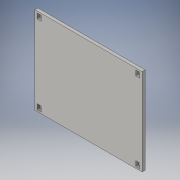
# Autodesk Inventor part: mcdave_top
Saved by Autodesk Inventor 2016 (Build 200138000, 138)
## iProperties
Created: 2017-11-29
Part Number: mcdave_top
Material: Generic
Document SubType Name: Modeling
Designer: student
Density: 1 g/cm^3
Appearance: Default
Author: student
Autodesk Inventor part; units mm, degrees
ref_plane "YZ Plane" through (0, 0, 0) normal (1, 0, 0) x (0, 1, 0)
ref_plane "XZ Plane" through (0, 0, 0) normal (0, 1, 0) x (-1, 0, 0)
ref_plane "XY Plane" through (0, 0, 0) normal (0, 0, 1) x (1, 0, 0)
sketch "Sketch1" plane through (0, 0, 0) normal (0, 0, 1) x (1, 0, 0)
  line L0 (49.1624, -46.1074) -> (-32.1176, -46.1074)
  line L1 (49.1624, -46.1074) -> (-32.1176, -46.1074)
  line L2 (-32.1176, -46.1074) -> (-32.1176, 19.9326)
  line L3 (-32.1176, -46.1074) -> (-32.1176, 19.9326)
  line L4 (49.1624, 19.9326) -> (-32.1176, 19.9326)
  line L5 (-32.1176, 19.9326) -> (49.1624, 19.9326)
  line L6 (49.1624, 19.9326) -> (49.1624, -46.1074)
  line L7 (44.3516, -40.9552) -> (47.5774, -40.9552)
  line L8 (44.3516, -40.9552) -> (47.5774, -40.9552)
  line L9 (47.5774, -40.9552) -> (47.5774, -44.8414)
  line L10 (47.5774, -40.9552) -> (47.5774, -44.8414)
  line L11 (47.5774, -44.8414) -> (44.3516, -44.8414)
  line L12 (47.5774, -44.8414) -> (44.3516, -44.8414)
  line L13 (44.3516, -44.8414) -> (44.3516, -40.9552)
  line L14 (44.3516, -44.8414) -> (44.3516, -40.9552)
  line L15 (47.5774, 14.7804) -> (47.5774, 18.6666)
  line L16 (47.5774, 14.7804) -> (44.3516, 14.7804)
  line L17 (44.3516, 14.7804) -> (44.3516, 18.6666)
  line L18 (44.3516, 14.7804) -> (44.3516, 18.6666)
  line L19 (44.3516, 18.6666) -> (47.5774, 18.6666)
  line L20 (44.3516, 18.6666) -> (47.5774, 18.6666)
  line L21 (47.5774, 18.6666) -> (47.5774, 14.7804)
  line L22 (-30.5326, -40.9421) -> (-27.3068, -40.9421)
  line L23 (-30.5326, -44.8414) -> (-27.3068, -44.8414)
  line L24 (-26.9875, -44.8414) -> (-30.5326, -44.8414)
  line L25 (-27.3068, 14.7804) -> (-30.5326, 14.7804)
  line L26 (-27.3068, 14.7804) -> (-30.5326, 14.7804)
  line L27 (-30.5326, 14.7804) -> (-30.5326, 18.6666)
  line L28 (-30.5326, 14.7804) -> (-30.5326, 18.6666)
  line L29 (-30.5326, 18.6666) -> (-27.3068, 18.6666)
  line L30 (-30.5326, 18.6666) -> (-27.3068, 18.6666)
  line L31 (-27.3068, 18.6666) -> (-27.3068, 14.7804)
  line L32 (-27.3068, 18.6666) -> (-27.3068, 14.7804)
  line L33 (-30.5326, -40.9421) -> (-30.5326, -44.8414)
  line L34 (-27.3068, -40.9421) -> (-27.3068, -44.8414)
  point P0 (0, 0)
  constraints: 71 end point, 9 collinear, 6 perpendicular, 3 horizontal, 1 vertical
extrude "Extrusion1" add sketch "Sketch1" along normal blind 2.286
body "Solid1"
